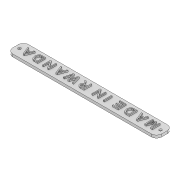
# Autodesk Inventor part: RWANDA_SIGN
Saved by Autodesk Inventor 2021 (Build 250183000, 183)
## iProperties
Created: 2021-12-15
Part Number: RWANDA_SIGN
Material: Generic
Document SubType Name: Modeling
Designer: Administrator
Density: 1 g/cm^3
Appearance: Default
Author: Administrator
Autodesk Inventor part; units mm, degrees
ref_plane "YZ Plane" through (0, 0, 0) normal (1, 0, 0) x (0, 1, 0)
ref_plane "XZ Plane" through (0, 0, 0) normal (0, 1, 0) x (-1, 0, 0)
ref_plane "XY Plane" through (0, 0, 0) normal (0, 0, 1) x (1, 0, 0)
sketch "Sketch1" plane through (0, 0, 0) normal (0, 1, 0) x (-1, 0, 0)
  line L0 (-298.1772, 27.7181) -> (276.1339, 27.7181) construction
  line L1 (276.1339, 27.7181) -> (276.1339, -22.2819) construction
  line L2 (276.1339, -22.2819) -> (-298.1772, -22.2819) construction
  line L3 (-298.1772, -22.2819) -> (-298.1772, 27.7181) construction
  line L4 (-295.0674, -2.2819) -> (-295.0674, 27.7181)
  line L5 (-295.0674, 27.7181) -> (-289.0995, 27.7181)
  line L6 (-289.0995, 27.7181) -> (-281.9882, 6.4757)
  spline S0 degree 2 poles (-281.9882, 6.4757) (-281.0049, 3.5031) (-280.5476, 2.0397) knots 0 0 0 1 1 1
  spline S1 degree 2 poles (-280.5476, 2.0397) (-280.0446, 3.6632) (-278.947, 6.8415) knots 0 0 0 1 1 1
  line L7 (-278.947, 6.8415) -> (-271.7443, 27.7181)
  line L8 (-271.7443, 27.7181) -> (-266.4165, 27.7181)
  line L9 (-266.4165, 27.7181) -> (-266.4165, -2.2819)
  line L10 (-266.4165, -2.2819) -> (-270.2351, -2.2819)
  line L11 (-270.2351, -2.2819) -> (-270.2351, 22.8248)
  line L12 (-270.2351, 22.8248) -> (-278.9927, -2.2819)
  line L13 (-278.9927, -2.2819) -> (-282.5598, -2.2819)
  line L14 (-282.5598, -2.2819) -> (-291.2488, 23.2592)
  line L15 (-291.2488, 23.2592) -> (-291.2488, -2.2819)
  line L16 (-291.2488, -2.2819) -> (-295.0674, -2.2819)
  line L17 (-251.6681, -2.2819) -> (-240.1437, 27.7181)
  line L18 (-240.1437, 27.7181) -> (-235.8449, 27.7181)
  line L19 (-235.8449, 27.7181) -> (-223.5888, -2.2819)
  line L20 (-223.5888, -2.2819) -> (-228.1162, -2.2819)
  line L21 (-228.1162, -2.2819) -> (-231.5918, 6.7958)
  line L22 (-231.5918, 6.7958) -> (-244.1681, 6.7958)
  line L23 (-244.1681, 6.7958) -> (-247.4607, -2.2819)
  line L24 (-247.4607, -2.2819) -> (-251.6681, -2.2819)
  line L25 (-243.0248, 10.0199) -> (-232.8266, 10.0199)
  line L26 (-232.8266, 10.0199) -> (-235.9821, 18.3431)
  spline S2 degree 2 poles (-235.9821, 18.3431) (-237.3998, 22.1388) (-238.0857, 24.5626) knots 0 0 0 1 1 1
  spline S3 degree 2 poles (-238.0857, 24.5626) (-238.6802, 21.6815) (-239.7092, 18.8233) knots 0 0 0 1 1 1
  line L27 (-239.7092, 18.8233) -> (-243.0248, 10.0199)
  line L28 (-208.7946, -2.2819) -> (-208.7946, 27.7181)
  line L29 (-208.7946, 27.7181) -> (-198.4592, 27.7181)
  spline S4 degree 2 poles (-198.4592, 27.7181) (-194.9607, 27.7181) (-193.1086, 27.2836) knots 0 0 0 1 1 1
  spline S5 degree 2 poles (-193.1086, 27.2836) (-190.5248, 26.6891) (-188.7184, 25.1342) knots 0 0 0 1 1 1
  spline S6 degree 2 poles (-188.7184, 25.1342) (-186.3403, 23.1449) (-183.9851, 16.9025) (-183.9851, 12.8781) knots 0 0 0 1 2 2 2
  spline S7 degree 2 poles (-183.9851, 12.8781) (-183.9851, 9.4711) (-185.5857, 4.1891) (-188.0781, 0.7364) (-191.0507, -1.253) (-195.2351, -2.2819) (-197.9562, -2.2819) knots 0 0 0 1 2 3 4 5 5 5
  line L30 (-197.9562, -2.2819) -> (-208.7946, -2.2819)
  line L31 (-204.8159, 1.2623) -> (-198.4135, 1.2623)
  spline S8 degree 2 poles (-198.4135, 1.2623) (-195.4409, 1.2623) (-192.0568, 2.3598) (-191.0735, 3.3659) knots 0 0 0 1 2 2 2
  spline S9 degree 2 poles (-191.0735, 3.3659) (-189.6559, 4.7836) (-188.0781, 9.5397) (-188.0781, 12.9467) knots 0 0 0 1 2 2 2
  spline S10 degree 2 poles (-188.0781, 12.9467) (-188.0781, 17.6571) (-191.165, 22.7105) (-193.383, 23.5565) knots 0 0 0 1 2 2 2
  spline S11 degree 2 poles (-193.383, 23.5565) (-194.9836, 24.1739) (-198.5049, 24.1739) knots 0 0 0 1 1 1
  line L32 (-198.5049, 24.1739) -> (-204.8159, 24.1739)
  line L33 (-204.8159, 24.1739) -> (-204.8159, 1.2623)
  line L34 (-166.79, -2.2819) -> (-166.79, 27.7181)
  line L35 (-166.79, 27.7181) -> (-145.0674, 27.7181)
  line L36 (-145.0674, 27.7181) -> (-145.0674, 24.1739)
  line L37 (-145.0674, 24.1739) -> (-162.8113, 24.1739)
  line L38 (-162.8113, 24.1739) -> (-162.8113, 15.0047)
  line L39 (-162.8113, 15.0047) -> (-146.1879, 15.0047)
  line L40 (-146.1879, 15.0047) -> (-146.1879, 11.4605)
  line L41 (-146.1879, 11.4605) -> (-162.8113, 11.4605)
  line L42 (-162.8113, 11.4605) -> (-162.8113, 1.2623)
  line L43 (-162.8113, 1.2623) -> (-144.3815, 1.2623)
  line L44 (-144.3815, 1.2623) -> (-144.3815, -2.2819)
  line L45 (-144.3815, -2.2819) -> (-166.79, -2.2819)
  line L46 (-114.9531, -2.2819) -> (-114.9531, 27.7181)
  line L47 (-114.9531, 27.7181) -> (-110.9745, 27.7181)
  line L48 (-110.9745, 27.7181) -> (-110.9745, -2.2819)
  line L49 (-110.9745, -2.2819) -> (-114.9531, -2.2819)
  line L50 (-92.3845, -2.2819) -> (-92.3845, 27.7181)
  line L51 (-92.3845, 27.7181) -> (-88.3144, 27.7181)
  line L52 (-88.3144, 27.7181) -> (-72.537, 4.1662)
  line L53 (-72.537, 4.1662) -> (-72.537, 27.7181)
  line L54 (-72.537, 27.7181) -> (-68.7412, 27.7181)
  line L55 (-68.7412, 27.7181) -> (-68.7412, -2.2819)
  line L56 (-68.7412, -2.2819) -> (-72.8113, -2.2819)
  line L57 (-72.8113, -2.2819) -> (-88.5888, 21.2699)
  line L58 (-88.5888, 21.2699) -> (-88.5888, -2.2819)
  line L59 (-88.5888, -2.2819) -> (-92.3845, -2.2819)
  line L60 (-38.7412, -2.2819) -> (-38.7412, 27.7181)
  line L61 (-38.7412, 27.7181) -> (-25.4333, 27.7181)
  spline S12 degree 2 poles (-25.4333, 27.7181) (-21.4318, 27.7181) (-17.2473, 26.0946) (-14.7549, 22.0016) (-14.7549, 19.5321) knots 0 0 0 1 2 3 3 3
  spline S13 degree 2 poles (-14.7549, 19.5321) (-14.7549, 16.3309) (-18.8937, 11.9635) (-23.1924, 11.369) knots 0 0 0 1 2 2 2
  spline S14 degree 2 poles (-23.1924, 11.369) (-21.6376, 10.6144) (-20.8144, 9.8827) knots 0 0 0 1 1 1
  spline S15 degree 2 poles (-20.8144, 9.8827) (-19.0766, 8.2821) (-17.5217, 5.8812) knots 0 0 0 1 1 1
  line L62 (-17.5217, 5.8812) -> (-12.3312, -2.2819)
  line L63 (-12.3312, -2.2819) -> (-17.2931, -2.2819)
  line L64 (-17.2931, -2.2819) -> (-21.2717, 3.9605)
  spline S16 degree 2 poles (-21.2717, 3.9605) (-23.0095, 6.6586) (-25.2504, 9.5169) (-27.0339, 10.683) (-27.9485, 10.9117) knots 0 0 0 1 2 3 3 3
  spline S17 degree 2 poles (-27.9485, 10.9117) (-28.6345, 11.0489) (-30.1665, 11.0489) knots 0 0 0 1 1 1
  line L65 (-30.1665, 11.0489) -> (-34.7626, 11.0489)
  line L66 (-34.7626, 11.0489) -> (-34.7626, -2.2819)
  line L67 (-34.7626, -2.2819) -> (-38.7412, -2.2819)
  line L68 (-34.7626, 14.4787) -> (-26.2336, 14.4787)
  spline S18 degree 2 poles (-26.2336, 14.4787) (-23.5126, 14.4787) (-20.4485, 15.5992) (-18.8479, 18.0915) (-18.8479, 19.5321) knots 0 0 0 1 2 3 3 3
  spline S19 degree 2 poles (-18.8479, 19.5321) (-18.8479, 21.6586) (-21.9348, 24.4025) (-25.2732, 24.4025) knots 0 0 0 1 2 2 2
  line L69 (-25.2732, 24.4025) -> (-34.7626, 24.4025)
  line L70 (-34.7626, 24.4025) -> (-34.7626, 14.4787)
  line L71 (8.3396, -2.2819) -> (0.3823, 27.7181)
  line L72 (0.3823, 27.7181) -> (4.4524, 27.7181)
  line L73 (4.4524, 27.7181) -> (9.0255, 8.0534)
  spline S20 degree 2 poles (9.0255, 8.0534) (9.7573, 4.9665) (10.306, 1.9025) knots 0 0 0 1 1 1
  spline S21 degree 2 poles (10.306, 1.9025) (11.4493, 6.7272) (11.6551, 7.4589) knots 0 0 0 1 1 1
  line L74 (11.6551, 7.4589) -> (17.3487, 27.7181)
  line L75 (17.3487, 27.7181) -> (22.1505, 27.7181)
  line L76 (22.1505, 27.7181) -> (26.4493, 12.5351)
  spline S22 degree 2 poles (26.4493, 12.5351) (28.0271, 6.8873) (28.7816, 1.9025) knots 0 0 0 1 1 1
  spline S23 degree 2 poles (28.7816, 1.9025) (29.3533, 4.7608) (30.2679, 8.4422) knots 0 0 0 1 1 1
  line L77 (30.2679, 8.4422) -> (34.9554, 27.7181)
  line L78 (34.9554, 27.7181) -> (38.9569, 27.7181)
  line L79 (38.9569, 27.7181) -> (30.771, -2.2819)
  line L80 (30.771, -2.2819) -> (26.8838, -2.2819)
  line L81 (26.8838, -2.2819) -> (20.6185, 20.5839)
  spline S24 degree 2 poles (20.6185, 20.5839) (19.7954, 23.4422) (19.6582, 24.1053) knots 0 0 0 1 1 1
  spline S25 degree 2 poles (19.6582, 24.1053) (19.1551, 22.0473) (18.7664, 20.5839) knots 0 0 0 1 1 1
  line L82 (18.7664, 20.5839) -> (12.4326, -2.2819)
  line L83 (12.4326, -2.2819) -> (8.3396, -2.2819)
  line L84 (51.0301, -2.2819) -> (62.5545, 27.7181)
  line L85 (62.5545, 27.7181) -> (66.8533, 27.7181)
  line L86 (66.8533, 27.7181) -> (79.1094, -2.2819)
  line L87 (79.1094, -2.2819) -> (74.5819, -2.2819)
  line L88 (74.5819, -2.2819) -> (71.1063, 6.7958)
  line L89 (71.1063, 6.7958) -> (58.5301, 6.7958)
  line L90 (58.5301, 6.7958) -> (55.2374, -2.2819)
  line L91 (55.2374, -2.2819) -> (51.0301, -2.2819)
  line L92 (59.6734, 10.0199) -> (69.8716, 10.0199)
  line L93 (69.8716, 10.0199) -> (66.7161, 18.3431)
  spline S26 degree 2 poles (66.7161, 18.3431) (65.2984, 22.1388) (64.6124, 24.5626) knots 0 0 0 1 1 1
  spline S27 degree 2 poles (64.6124, 24.5626) (64.0179, 21.6815) (62.989, 18.8233) knots 0 0 0 1 1 1
  line L94 (62.989, 18.8233) -> (59.6734, 10.0199)
  line L95 (93.8807, -2.2819) -> (93.8807, 27.7181)
  line L96 (93.8807, 27.7181) -> (97.9508, 27.7181)
  line L97 (97.9508, 27.7181) -> (113.7283, 4.1662)
  line L98 (113.7283, 4.1662) -> (113.7283, 27.7181)
  line L99 (113.7283, 27.7181) -> (117.524, 27.7181)
  line L100 (117.524, 27.7181) -> (117.524, -2.2819)
  line L101 (117.524, -2.2819) -> (113.4539, -2.2819)
  line L102 (113.4539, -2.2819) -> (97.6765, 21.2699)
  line L103 (97.6765, 21.2699) -> (97.6765, -2.2819)
  line L104 (97.6765, -2.2819) -> (93.8807, -2.2819)
  line L105 (135.8167, -2.2819) -> (135.8167, 27.7181)
  line L106 (135.8167, 27.7181) -> (146.1521, 27.7181)
  spline S28 degree 2 poles (146.1521, 27.7181) (149.6505, 27.7181) (151.5027, 27.2836) knots 0 0 0 1 1 1
  spline S29 degree 2 poles (151.5027, 27.2836) (154.0865, 26.6891) (155.8929, 25.1342) knots 0 0 0 1 1 1
  spline S30 degree 2 poles (155.8929, 25.1342) (158.271, 23.1449) (160.6262, 16.9025) (160.6262, 12.8781) knots 0 0 0 1 2 2 2
  spline S31 degree 2 poles (160.6262, 12.8781) (160.6262, 9.4711) (159.0255, 4.1891) (156.5332, 0.7364) (153.5606, -1.253) (149.3762, -2.2819) (146.6551, -2.2819) knots 0 0 0 1 2 3 4 5 5 5
  line L107 (146.6551, -2.2819) -> (135.8167, -2.2819)
  line L108 (139.7954, 1.2623) -> (146.1978, 1.2623)
  spline S32 degree 2 poles (146.1978, 1.2623) (149.1704, 1.2623) (152.5545, 2.3598) (153.5377, 3.3659) knots 0 0 0 1 2 2 2
  spline S33 degree 2 poles (153.5377, 3.3659) (154.9554, 4.7836) (156.5332, 9.5397) (156.5332, 12.9467) knots 0 0 0 1 2 2 2
  spline S34 degree 2 poles (156.5332, 12.9467) (156.5332, 17.6571) (153.4463, 22.7105) (151.2283, 23.5565) knots 0 0 0 1 2 2 2
  spline S35 degree 2 poles (151.2283, 23.5565) (149.6277, 24.1739) (146.1063, 24.1739) knots 0 0 0 1 1 1
  line L109 (146.1063, 24.1739) -> (139.7954, 24.1739)
  line L110 (139.7954, 24.1739) -> (139.7954, 1.2623)
  line L111 (174.46, -2.2819) -> (185.9844, 27.7181)
  line L112 (185.9844, 27.7181) -> (190.2832, 27.7181)
  line L113 (190.2832, 27.7181) -> (202.5393, -2.2819)
  line L114 (202.5393, -2.2819) -> (198.0118, -2.2819)
  line L115 (198.0118, -2.2819) -> (194.5362, 6.7958)
  line L116 (194.5362, 6.7958) -> (181.96, 6.7958)
  line L117 (181.96, 6.7958) -> (178.6673, -2.2819)
  line L118 (178.6673, -2.2819) -> (174.46, -2.2819)
  line L119 (183.1033, 10.0199) -> (193.3015, 10.0199)
  line L120 (193.3015, 10.0199) -> (190.146, 18.3431)
  spline S36 degree 2 poles (190.146, 18.3431) (188.7283, 22.1388) (188.0423, 24.5626) knots 0 0 0 1 1 1
  spline S37 degree 2 poles (188.0423, 24.5626) (187.4478, 21.6815) (186.4188, 18.8233) knots 0 0 0 1 1 1
  line L121 (186.4188, 18.8233) -> (183.1033, 10.0199)
  point P0 (0, 0)
  dimension "d0" = 574.3111
  constraints: 2 other
  measures "d0" distance of L1.end L2.end
extrude "Extrusion1" add sketch "Sketch1" along normal blind 5
sketch "Sketch2" plane through (0, 0, 0) normal (0, -1, 0) x (1, 0, 0)
  line L0 (-190.2832, 27.7181) -> (-202.5393, -2.2819) projected
  line L1 (-233.7358, -17.2819) -> (326.2642, -17.2819)
  line L2 (326.2642, -17.2819) -> (326.2642, 42.7181)
  line L3 (326.2642, 42.7181) -> (-233.7358, 42.7181)
  line L4 (-233.7358, 42.7181) -> (-233.7358, -17.2819)
  line L5 (-233.7358, -17.2819) -> (326.2642, 42.7181) construction
  line L6 (326.2642, -17.2819) -> (-233.7358, 42.7181) construction
  line L7 (282.5598, -2.2819) -> (282.1898, -3.3696) projected
  point P0 (0, 0)
  point P1 (46.2642, 12.7181)
  point P2 (282.5598, -2.2819)
  point P3 (278.9927, -2.2819)
  point P4 (295.0674, -2.2819)
  dimension "d3" = 560
  dimension "d4" = 60
  dimension "d11" = 31.1965
  dimension "d12" = 15
  constraints: 12 end point, 2 midpoint, 2 parallel, 1 horizontal, 1 perpendicular
  measures "d3" distance of L3.end L2.end
  measures "d4" distance of L2.end L1.end
  measures "d11" distance from line of L4 L0.end
extrude "Extrusion2" add sketch "Sketch2" along normal blind 10
fillet "Fillet2" radius 20 4 edges at (326.2642, -5, -17.2819) (-233.7358, -5, -17.2819) (-233.7358, -5, 42.7181) (326.2642, -5, 42.7181)
sketch "Sketch3" plane through (0, 0, 0) normal (0, 1, 0) x (1, 0, 0)
  line L0 (326.2642, -2.7181) -> (326.2642, -22.7181) projected
  line L1 (-233.7358, -22.7181) -> (-233.7358, -2.7181) projected
  point P0 (0, 0)
  point P1 (311.2642, -12.7181)
  point P2 (-218.7358, -12.7181)
  dimension "d14" = 15
  dimension "d15" = 15
  measures "d14" distance from line of L0 point (311.264, -12.718)
  measures "d15" distance from line of L1 point (-218.736, -12.718)
hole "Hole1" at (311.2642, 0, 12.7181) at (-218.7358, 0, 12.7181) direction (0, -1, 0) diameter 5.5 end through all countersink diameter 10.4 countersink angle 90 clearance for "Countersunk Flat Head Screw ISO 2009/7046" size "M5" standard "ISO"
body "Solid1"
